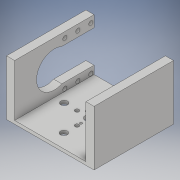
# Autodesk Inventor part: база захвата
Saved by Autodesk Inventor 2019 (Build 230136000, 136)
## iProperties
Created: 2019-08-15
Part Number: база захвата
Material: Типовые
Document SubType Name: Modeling
Designer: Петров Иван
Density: 1 g/cm^3
Appearance: По умолчанию
Author: Петров Иван
Autodesk Inventor part; units mm, degrees
ref_plane "YZ Plane" through (0, 0, 0) normal (1, 0, 0) x (0, 1, 0)
ref_plane "XZ Plane" through (0, 0, 0) normal (0, 1, 0) x (-1, 0, 0)
ref_plane "XY Plane" through (0, 0, 0) normal (0, 0, 1) x (1, 0, 0)
sketch "Эскиз1" plane through (0, 0, 0) normal (0, 1, 0) x (-1, 0, 0)
  circle A0 centre (15.9998, -0.0856) radius 2.1
  circle A1 centre (-15.9998, 0.0856) radius 2.1
  circle A2 centre (0.0856, 15.9998) radius 2.1
  circle A3 centre (-0.0856, -15.9998) radius 2.1
  circle A4 centre (0, 0) radius 2.9
  circle A5 centre (8, 0) radius 1.25
  circle A6 centre (0, 8) radius 1.25
  circle A7 centre (-8, 0) radius 1.25
  circle A8 centre (4.7631, -2.75) radius 0.75
  circle A9 centre (-4.7631, -2.75) radius 0.75
  circle A10 centre (0, 5.5) radius 0.75
  circle A11 centre (0, -8) radius 1.25
  circle A12 centre (0, 0) radius 24.5
  line L0 (27, -24.5) -> (-27, -24.5)
  line L1 (-27, -24.5) -> (-27, 24.5)
  line L2 (-27, 24.5) -> (27, 24.5)
  line L3 (27, 24.5) -> (27, -24.5)
  line L4 (27, -24.5) -> (-27, 24.5) construction
  line L5 (-27, -24.5) -> (27, 24.5) construction
  dimension "d22" = 54
  dimension "d23" = 49
  constraints: 13 centre point, 12 end point, 2 midpoint, 2 parallel, 1 horizontal, 1 perpendicular
  measures "d22" distance of L1.end L2.end
  measures "d23" distance of L0.end L1.end
extrude "Выдавливание1" add sketch "Эскиз1" along normal blind 2
sketch "Эскиз8" plane through (0, 2, 0) normal (0, 1, 0) x (1, 0, 0)
  line L0 (27, -24.5) -> (27, 24.5) projected
  line L1 (-27, -24.5) -> (27, -24.5) projected
  line L2 (27, 24.5) -> (22, 24.5)
  line L3 (22, 24.5) -> (22, -24.5)
  line L4 (22, -24.5) -> (27, -24.5)
  line L5 (27, -24.5) -> (27, 24.5)
  line L6 (-27, -24.5) -> (-22, -24.5)
  line L7 (-22, -24.5) -> (-22, 24.5)
  line L8 (-22, 24.5) -> (-27, 24.5)
  line L9 (-27, 24.5) -> (-27, -24.5)
  point P0 (0, 0)
  dimension "d24" = 5
  dimension "d25" = 5
  constraints: 16 end point, 4 parallel, 2 horizontal, 2 perpendicular, 1 point on line
  measures "d24" distance of L4.end L3.end
  measures "d25" distance of L8.end L7.end
extrude "Выдавливание7" add sketch "Эскиз8" along normal blind 32
sketch "Эскиз9" plane through (-27, 0, -24.5) normal (-1, 0, 0) x (0, 0, 1)
  line L0 (6.7, 29.6) -> (6.7, 31.9)
  line L1 (6.7, 29.6) -> (5.3, 29.6)
  line L2 (5.3, 31.9) -> (5.3, 29.6)
  line L3 (-1.3, 31.9) -> (5.3, 31.9)
  line L4 (-1.3, 29.6) -> (-1.3, 31.9)
  circle A0 centre (24.5, 17) radius 9.15
  circle A1 centre (24.5, 17) radius 1.5
  circle A2 centre (-11.5, 9) radius 1.3
  circle A3 centre (2, 3.5) radius 1.3
  circle A4 centre (-6, 3.5) radius 1.3
  circle A5 centre (10, 3.5) radius 1.3
  circle A6 centre (18, 3.5) radius 1.3
  circle A7 centre (-11.5, 25) radius 1.3
  circle A8 centre (2, 30.5) radius 1.3
  circle A9 centre (-6, 30.5) radius 1.3
  circle A10 centre (10, 30.5) radius 1.3
  circle A11 centre (18, 30.5) radius 1.3
  line L5 (35.5198, 17.1) -> (34.9796, 17.1)
  line L6 (35.5198, 24) -> (35.5198, 17.1)
  arc A12 (35.5198, 24) -> (35.4686, 24.75) centre (30, 24) ccw
  line L7 (33, 24.75) -> (35.4686, 24.75)
  arc A13 (31.25, 26.5) -> (33, 24.75) centre (33, 26.5) ccw
  line L8 (31.25, 27) -> (31.25, 26.5)
  line L9 (-6.3063, 27) -> (31.25, 27)
  arc A14 (-6.3063, 27) -> (-6.9945, 26.6078) centre (-6.3063, 26.2) ccw
  arc A15 (-6.9945, 26.6078) -> (-7.6078, 25.9945) centre (-8.5, 27.5) ccw
  arc A16 (-7.6078, 25.9945) -> (-8, 25.3063) centre (-7.2, 25.3063) ccw
  line L10 (-8, 8.6937) -> (-8, 25.3063)
  arc A17 (-8, 8.6937) -> (-7.6078, 8.0055) centre (-7.2, 8.6937) ccw
  arc A18 (-6.9945, 7.3922) -> (-7.6078, 8.0055) centre (-8.5, 6.5) ccw
  arc A19 (-7.6078, 8.0055) -> (-6.9945, 7.3922) centre (-8.5, 6.5) ccw
  line L11 (31.25, 28.3229) -> (31.25, 27)
  arc A20 (31.25, 28.3229) -> (30, 28.5) centre (29.9989, 23.9922) ccw
  line L12 (30, 28.5) -> (22.5, 28.5)
  line L13 (22.5, 29.6) -> (22.5, 28.5)
  line L14 (21.3, 29.6) -> (22.5, 29.6)
  line L15 (21.3, 31.9) -> (21.3, 29.6)
  line L16 (14.7, 31.9) -> (21.3, 31.9)
  line L17 (14.7, 29.6) -> (14.7, 31.9)
  line L18 (13.3, 29.6) -> (14.7, 29.6)
  line L19 (13.3, 31.9) -> (13.3, 29.6)
  line L20 (6.7, 31.9) -> (13.3, 31.9)
  line L21 (6.7, 29.6) -> (6.7, 31.9)
  line L22 (5.3, 29.6) -> (6.7, 29.6)
  line L23 (5.3, 31.9) -> (5.3, 29.6)
  line L24 (-1.3, 31.9) -> (5.3, 31.9)
  line L25 (-1.3, 29.6) -> (-1.3, 31.9)
  line L26 (-2.7, 29.6) -> (-1.3, 29.6)
  line L27 (-2.7, 31.9) -> (-2.7, 29.6)
  line L28 (-9.3, 31.9) -> (-2.7, 31.9)
  line L29 (-9.3, 29.6) -> (-9.3, 31.9)
  line L30 (-10.5198, 29.6) -> (-9.3, 29.6)
  arc A21 (-10.5198, 29.6) -> (-10.6, 29.5198) centre (-9.5, 28.5) ccw
  line L31 (-10.6, 28.3) -> (-10.6, 29.5198)
  line L32 (-12.9, 28.3) -> (-10.6, 28.3)
  line L33 (-12.9, 21.7) -> (-12.9, 28.3)
  line L34 (-10.6, 21.7) -> (-12.9, 21.7)
  line L35 (-10.6, 12.3) -> (-10.6, 21.7)
  line L36 (-12.9, 12.3) -> (-10.6, 12.3)
  line L37 (-12.9, 5.7) -> (-12.9, 12.3)
  line L38 (-10.6, 5.7) -> (-12.9, 5.7)
  line L39 (-10.6, 4.4802) -> (-10.6, 5.7)
  arc A22 (-10.6, 4.4802) -> (-10.5198, 4.4) centre (-9.5, 5.5) ccw
  line L40 (-9.3, 4.4) -> (-10.5198, 4.4)
  line L41 (-9.3, 2.1) -> (-9.3, 4.4)
  line L42 (-2.7, 2.1) -> (-9.3, 2.1)
  line L43 (-2.7, 4.4) -> (-2.7, 2.1)
  line L44 (-1.3, 4.4) -> (-2.7, 4.4)
  line L45 (-1.3, 2.1) -> (-1.3, 4.4)
  line L46 (5.3, 2.1) -> (-1.3, 2.1)
  line L47 (5.3, 4.4) -> (5.3, 2.1)
  line L48 (6.7, 4.4) -> (5.3, 4.4)
  line L49 (6.7, 2.1) -> (6.7, 4.4)
  line L50 (13.3, 2.1) -> (6.7, 2.1)
  line L51 (13.3, 4.4) -> (13.3, 2.1)
  line L52 (14.7, 4.4) -> (13.3, 4.4)
  line L53 (14.7, 2.1) -> (14.7, 4.4)
  line L54 (21.3, 2.1) -> (14.7, 2.1)
  line L55 (21.3, 4.4) -> (21.3, 2.1)
  line L56 (22.5, 4.4) -> (21.3, 4.4)
  line L57 (22.5, 5.5) -> (22.5, 4.4)
  line L58 (30, 5.5) -> (22.5, 5.5)
  arc A23 (30, 5.5) -> (31.25, 5.6771) centre (29.9989, 10.0078) ccw
  line L59 (31.25, 7) -> (31.25, 5.6771)
  line L60 (31.25, 7.5) -> (31.25, 7)
  arc A24 (33, 9.25) -> (31.25, 7.5) centre (33, 7.5) ccw
  line L61 (35.4686, 9.25) -> (33, 9.25)
  arc A25 (35.4686, 9.25) -> (35.5198, 10) centre (30, 10) ccw
  line L62 (35.5198, 16.9) -> (35.5198, 10)
  line L63 (34.9796, 16.9) -> (35.5198, 16.9)
  arc A26 (-7.6078, 25.9945) -> (-6.9945, 26.6078) centre (-8.5, 27.5) ccw
  arc A27 (-6.9945, 7.3922) -> (-6.3063, 7) centre (-6.3063, 7.8) ccw
  line L64 (31.25, 7) -> (-6.3063, 7)
  line L65 (0, 0) -> (0, 34) projected
  line L66 (0, 0) -> (24.5, 0)
  line L67 (24.5, 0) -> (24.5, 15.5)
  line L68 (24.5, 17) -> (23, 17)
  line L69 (0, 7) -> (0, 0)
  line L70 (24.5, 26.15) -> (24.5, 27)
  line L71 (24.5, 7.85) -> (24.5, 7)
  dimension "d28" = 17
  constraints: 142 end point, 36 point on circle, 28 centre point, 5 point on line, 2 parallel, 2 perpendicular, 1 horizontal
  measures "d28" distance of L68.start L66.end
extrude "Выдавливание8" cut sketch "Эскиз9" against normal blind 5 contours L65 L64 A27 A18 A17 L10 A16 A26 A14 L9 | L9 L70 A0 L67 L64 L65 | A0 | A1 | A3 | A5 | A6 | A8 | A10 | A11
sketch "Эскиз10" plane through (-27, 0, -24.5) normal (-1, 0, 0) x (0, 0, 1)
  arc A0 (24.5, 7.85) -> (24.5, 26.15) centre (24.5, 17) ccw projected
  circle A1 centre (24.5, 17) radius 11
  point P0 (24.5, 0)
  dimension "d31" = 22
  constraints: 1 centre point, 1 coincident
  measures "d31" diameter of A1
extrude "Выдавливание9" cut sketch "Эскиз10" against normal blind 5
